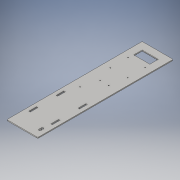
# Autodesk Inventor part: Board Cage 2
Saved by Autodesk Inventor 2016 (Build 200138000, 138)
## iProperties
Created: 2017-09-11
Part Number: Board Cage 2
Material: Generic
Document SubType Name: Modeling
Designer: Student
Density: 1 g/cm^3
Appearance: Default
Author: Student
Autodesk Inventor part; units mm, degrees
ref_plane "YZ Plane" through (0, 0, 0) normal (1, 0, 0) x (0, 1, 0)
ref_plane "XZ Plane" through (0, 0, 0) normal (0, 1, 0) x (-1, 0, 0)
ref_plane "XY Plane" through (0, 0, 0) normal (0, 0, 1) x (1, 0, 0)
sketch "Sketch1" plane through (0, 0, 0) normal (0, 1, 0) x (-1, 0, 0)
  line L0 (0, 0) -> (0, -444.5)
  line L1 (0, -444.5) -> (101.6, -444.5)
  line L2 (101.6, -444.5) -> (101.6, 0)
  line L3 (101.6, 0) -> (0, 0)
  dimension "d0" = 444.5
  dimension "d1" = 101.6
  constraints: 8 end point, 2 perpendicular, 1 horizontal, 1 vertical
  measures "d0" distance of L0.start L0.end
  measures "d1" distance of L0.end L1.end
extrude "Extrusion1" add sketch "Sketch1" along normal blind 3.175
sketch "Sketch2" plane through (0, 3.175, 0) normal (0, 1, 0) x (1, 0, 0)
  line L0 (0, 444.5) -> (-101.6, 444.5) projected
  line L1 (-101.6, 444.5) -> (-101.6, 419.1)
  line L2 (-76.2, 419.1) -> (-76.2, 393.7)
  line L3 (-101.6, 0) -> (0, 0) projected
  line L4 (-50.8, 0) -> (-50.8, 463.567) construction
  line L5 (0, 444.5) -> (0, 419.1)
  line L6 (-25.4, 419.1) -> (-25.4, 393.7)
  line L7 (-101.6, 393.7) -> (-101.6, 0)
  line L8 (-101.6, 0) -> (0, 0)
  line L9 (0, 393.7) -> (0, 0)
  line L10 (-76.2, 393.7) -> (-25.4, 393.7)
  line L11 (-76.2, 419.1) -> (-25.4, 419.1)
  line L12 (-101.6, 444.5) -> (-101.6, 0) projected
  dimension "d6" = 25.4
  dimension "d46" = 25.4
  dimension "d47" = 25.4
  constraints: 20 end point, 4 symmetric about line, 2 equal length, 2 perpendicular, 2 point on line, 2 vertical, 1 midpoint
  measures "d6" distance of L2.start L2.end
  measures "d46" distance between parallel lines of L0 L11
  measures "d47" distance between parallel lines of L12 L2
extrude "Extrusion2" cut sketch "Sketch2" against normal blind 3.175
sketch "Sketch3" plane through (0, 3.175, 0) normal (0, 1, 0) x (1, 0, 0)
  line L0 (0, 444.5) -> (-101.6, 444.5) projected
  line L1 (-50.8, 444.5) -> (-50.8, -69.4552) construction
  line L2 (-50.8, 375.5095) -> (-79.0575, 375.5095) construction
  line L3 (-79.0575, 375.5095) -> (-79.0575, 317.5095) construction
  line L4 (-50.8, 375.5095) -> (-22.5425, 375.5095) construction
  line L5 (-22.5425, 375.5095) -> (-22.5425, 317.5095) construction
  line L6 (-79.0575, 317.5095) -> (-22.5425, 317.5095) construction
  circle A0 centre (-79.0575, 317.5095) radius 1.5
  circle A1 centre (-22.5425, 317.5095) radius 1.5
  circle A2 centre (-22.5425, 375.5095) radius 1.5
  circle A3 centre (-79.0575, 375.5095) radius 1.5
  point P0 (0, 0)
  dimension "d9" = 28.2575
  dimension "d10" = 58
  dimension "d11" = 3
  constraints: 12 end point, 4 centre point, 4 coincident, 2 horizontal, 2 symmetric about line, 2 vertical, 1 midpoint, 1 point on line
  measures "d9" distance of L2.start L2.end
  measures "d10" distance of L2.end L3.end
  measures "d11" diameter of A0
hole "Hole1" at (-79.0575, 3.175, -317.5095) at (-22.5425, 3.175, -317.5095) at (-79.0575, 3.175, -375.5095) at (-22.5425, 3.175, -375.5095) direction (0, -1, 0) diameter 3 end through all
sketch "Sketch4" plane through (0, 3.175, 0) normal (0, 1, 0) x (1, 0, 0)
  line L0 (0, 444.5) -> (-101.6, 444.5) projected
  line L1 (-50.8, 444.5) -> (-50.8, -14.5514) construction
  line L2 (-50.8, 266.7) -> (-77.3, 266.7) construction
  line L3 (-77.3, 266.7) -> (-77.3, 198.7) construction
  line L4 (-77.3, 198.7) -> (-50.8, 198.7) construction
  line L5 (-50.8, 266.7) -> (-24.3, 266.7) construction
  line L6 (-24.3, 266.7) -> (-24.3, 198.7) construction
  line L7 (-24.3, 198.7) -> (-50.8, 198.7) construction
  circle A0 centre (-74.8, 213.7) radius 1.5
  circle A1 centre (-31.3, 264.2) radius 1.5
  circle A2 centre (-59.3, 264.2) radius 1.5
  point P0 (0, 0)
  dimension "d19" = 26.5
  dimension "d20" = 68
  dimension "d21" = 3
  dimension "d22" = 15
  dimension "d23" = 50.5
  dimension "d24" = 3
  dimension "d25" = 3
  dimension "d26" = 7
  dimension "d27" = 65.5
  dimension "d28" = 35
  dimension "d29" = 65.5
  dimension "d37" = 177.8
  constraints: 14 end point, 3 centre point, 2 point on line, 2 symmetric about line, 2 vertical, 1 horizontal, 1 midpoint, 1 perpendicular
  measures "d19" distance of L2.start L2.end
  measures "d20" distance of L2.end L3.end
  measures "d21" diameter of A0
  measures "d22" distance from line of L4 A0.centre
  measures "d23" distance from line of L6 A0.centre
  measures "d24" diameter of A1
  measures "d25" diameter of A2
  measures "d26" distance from line of L6 A1.centre
  measures "d27" distance from line of L7 A1.centre
  measures "d28" horizontal distance of L6.start A2.centre
  measures "d29" distance from line of L4 A2.centre
  measures "d37" distance between parallel lines of L2 L0
hole "Hole2" at (-74.8, 3.175, -213.7) at (-59.3, 3.175, -264.2) at (-31.3, 3.175, -264.2) direction (0, -1, 0) diameter 3 end through all
sketch "Sketch5" plane through (0, 3.175, 0) normal (0, 1, 0) x (1, 0, 0)
  line L0 (-101.6, 0) -> (0, 0) projected
  line L1 (-50.8, 0) -> (-50.8, 459.8943) construction
  line L2 (-50.8, 203.2) -> (-84.455, 203.2)
  line L3 (-84.455, 203.2) -> (-84.455, 31.75)
  line L4 (0, 444.5) -> (-101.6, 444.5) projected
  line L5 (-50.8, 203.2) -> (-17.145, 203.2)
  line L6 (-17.145, 203.2) -> (-17.145, 31.75)
  line L7 (-84.455, 31.75) -> (-17.145, 31.75)
  line L8 (-84.455, 59.8594) -> (-84.455, 85.2594)
  line L9 (-84.455, 85.2594) -> (-89.455, 85.2594)
  line L10 (-89.455, 85.2594) -> (-89.455, 59.8594)
  line L11 (-89.455, 59.8594) -> (-84.455, 59.8594)
  line L12 (-84.455, 117.475) -> (-17.145, 117.475) construction
  line L13 (-17.145, 59.8594) -> (-17.145, 85.2594)
  line L14 (-17.145, 85.2594) -> (-12.145, 85.2594)
  line L15 (-12.145, 85.2594) -> (-12.145, 59.8594)
  line L16 (-12.145, 59.8594) -> (-17.145, 59.8594)
  line L17 (-17.145, 117.475) -> (-84.455, 117.475) construction
  line L18 (-84.455, 175.0906) -> (-84.455, 149.6906)
  line L19 (-84.455, 149.6906) -> (-89.455, 149.6906)
  line L20 (-89.455, 149.6906) -> (-89.455, 175.0906)
  line L21 (-89.455, 175.0906) -> (-84.455, 175.0906)
  line L22 (-17.145, 149.6906) -> (-12.145, 149.6906)
  line L23 (-17.145, 175.0906) -> (-17.145, 149.6906)
  line L24 (-12.145, 175.0906) -> (-17.145, 175.0906)
  line L25 (-12.145, 149.6906) -> (-12.145, 175.0906)
  dimension "d38" = 33.655
  dimension "d39" = 171.45
  dimension "d40" = 241.3
  dimension "d41" = 25.4
  dimension "d42" = 5
  constraints: 48 end point, 16 symmetric about line, 3 midpoint, 3 perpendicular, 3 point on line, 2 horizontal, 1 parallel, 1 vertical
  measures "d38" distance of L2.start L2.end
  measures "d39" distance of L2.end L3.end
  measures "d40" distance between parallel lines of L4 L2
  measures "d41" distance of L8.start L8.end
  measures "d42" distance of L8.end L9.end
extrude "Extrusion3" cut sketch "Sketch5" against normal blind 3.175 contours L3 L19 L20 L21 | L24 L25 L22 L6 | L3 L11 L10 L9 | L14 L15 L16 L6
sketch "Sketch6" plane through (0, 3.175, 0) normal (0, 1, 0) x (1, 0, 0)
  circle A0 centre (-18.1376, 25.4) radius 3.81
  circle A1 centre (-18.1376, 33.02) radius 3.81
  line L0 (-101.6, 0) -> (0, 0) projected
  dimension "d48" = 7.62
  dimension "d49" = 7.62
  dimension "d57" = 25.4
  dimension "d58" = 33.02
  constraints: 2 centre point
  measures "d48" diameter of A0
  measures "d49" diameter of A1
  measures "d57" distance from line of L0 A0.centre
  measures "d58" distance from line of L0 A1.centre
hole "Hole3" at (-18.1376, 3.175, -33.02) at (-18.1376, 3.175, -25.4) direction (0, -1, 0) diameter 7.62 end through all
fillet "Fillet1" radius 3.175 3 edges at (0, 1.5875, -444.5) (-101.6, 1.5875, 0) (0, 1.5875, 0)
fillet "Fillet2" radius 3.175 1 edges at (-101.6, 1.5875, -444.5)
fillet "Fillet3" radius 1.27 8 edges at (-50.8, 0, -393.7) (-50.8, 3.175, -393.7) (-25.4, 0, -406.4) (-25.4, 3.175, -406.4) (-50.8, 3.175, -419.1) (-76.2, 3.175, -406.4) (-76.2, 0, -406.4) (-50.8, 0, -419.1)
body "Solid1"
